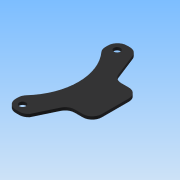
# Autodesk Inventor part: крепление вентилятора1
Saved by Autodesk Inventor 2017 (Build 210142000, 142)
## iProperties
Part Number: крепление вентилятора1
Material: Типовые
Document SubType Name: Modeling
Designer: Max
Mass: 1.88461 g
Surface Area: 28.4588 cm^2
Volume: 1.88461 cm^3
Density: 1 g/cm^3
Appearance: Резина — черная
Author: Max
Autodesk Inventor part; units mm, degrees
ref_plane "YZ Plane" through (0, 0, 0) normal (1, 0, 0) x (0, 1, 0)
ref_plane "XZ Plane" through (0, 0, 0) normal (0, 1, 0) x (-1, 0, 0)
ref_plane "XY Plane" through (0, 0, 0) normal (0, 0, 1) x (1, 0, 0)
sketch "Эскиз1" plane through (0, 0, 0) normal (0, 0, 1) x (1, 0, 0)
  circle A0 centre (25, -25) radius 1.75
  circle A1 centre (25, 25) radius 1.75
  line L0 (20.6111, 32.2931) -> (30.5924, 32.2931)
  line L1 (30.4739, -29.2685) -> (20.6111, -29.2685)
  line L2 (40.1458, 7.8878) -> (58.5047, 7.8878)
  line L3 (58.5047, 7.8878) -> (58.5047, -21.7573)
  line L4 (58.5047, -21.7573) -> (34.0362, -21.7573)
  arc A2 (29.5, 0) -> (20.6111, 21.1053) centre (0, 0) ccw
  arc A3 (20.6111, -21.1053) -> (29.5, 0) centre (0, 0) ccw
  line L5 (30.5924, 32.2931) -> (40.1458, 7.8878)
  line L6 (30.4739, -29.2685) -> (34.0362, -21.7573)
  line L7 (20.6111, -29.2685) -> (20.6111, -21.1053)
  line L8 (20.6111, 21.1053) -> (20.6111, 32.2931)
  line L9 (25, 25) -> (25, -25) construction
  line L10 (25, 0) -> (58.5047, 0) construction
  dimension "d10" = 25
  dimension "d11" = 25
  constraints: 22 end point, 4 centre point, 4 point on circle, 1 midpoint, 1 perpendicular, 1 point on line, 1 vertical
  measures "d10" distance from line of L10 L9.end
  measures "d11" distance from line of L10 L9.start
extrude "Выдавливание1" add sketch "Эскиз1" along normal blind 1.5
fillet "Сопряжение1" radius 5 10 edges at (20.6111, -29.2685, 0.75) (20.6111, 32.2931, 0.75) (20.6111, -21.1053, 0.75) (20.6111, 21.1053, 0.75) (30.5924, 32.2931, 0.75) (40.1458, 7.8878, 0.75) (34.0362, -21.7573, 0.75) (58.5047, -21.7573, 0.75) (58.5047, 7.8878, 0.75) (30.4739, -29.2685, 0.75)
sketch "Эскиз2" plane through (0, 0, 1.5) normal (0, 0, 1) x (1, 0, 0)
  line L0 (55.5047, 2.0132) -> (55.5047, -17.9868)
  line L1 (55.5047, -17.9868) -> (55.5047, 2.0132)
  circle A0 centre (55.5047, 2.0132) radius 1.5
  circle A1 centre (55.5047, -17.9868) radius 1.5
  line L2 (58.5047, 2.8878) -> (58.5047, -16.7573) projected
  line L3 (58.5047, -16.7573) -> (58.5047, 2.8878) projected
  line L4 (58.5047, -7.9868) -> (55.5047, -7.9868)
  point P0 (0, 0)
  dimension "d4" = 3
  dimension "d5" = 3
  dimension "d6" = 3
  dimension "d7" = 20
  constraints: 6 end point, 2 centre point, 2 coincident, 1 collinear, 1 midpoint, 1 perpendicular, 1 point on line, 1 symmetric about line, 1 vertical
  measures "d4" diameter of A0
  measures "d5" diameter of A1
  measures "d6" distance between parallel lines of L2 L0
  measures "d7" distance of L0.end L0.start
extrude "Выдавливание2" cut sketch "Эскиз2" against normal blind 1.5
